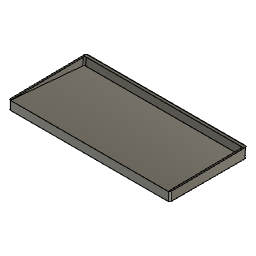
Resistor Stand v4 (Autodesk Fusion 360 design; units mm, degrees)
Autodesk Fusion 360 part; units mm, degrees
sketch "Sketch1" plane through (0, 0, 0) normal (1, 0, 0) x (0, 1, 0)
  line L0 (0, 0) -> (0, 5.5344)
  line L1 (0, 5.5344) -> (63.2584, 0)
  line L2 (63.2584, 0) -> (63.8118, 6.3258)
  line L3 (63.8118, 6.3258) -> (61.2815, 6.5472) construction
  line L4 (61.2815, 6.5472) -> (60.728, 0.2214) construction
  line L5 (0, 0) -> (63.2584, 0) construction
  line L6 (63.2584, 0) -> (63.2584, -1.905) construction
  line L7 (63.2584, -1.905) -> (0, -1.905)
  line L8 (0, -1.905) -> (0, 0)
  line L9 (66.3421, 6.1045) -> (65.7887, -0.2214)
  line L10 (63.8118, 6.3258) -> (66.3421, 6.1045) construction
  line L11 (63.2584, 0) -> (65.8081, 0) construction
  line L12 (65.8081, 0) -> (65.8081, -1.905)
  line L13 (65.8081, -1.905) -> (63.2584, -1.905)
  line L14 (63.8118, 6.3258) -> (66.3421, 6.1045) construction
  line L15 (63.8118, 6.3258) -> (66.3421, 6.3258)
  line L16 (66.3421, 6.3258) -> (66.3421, 6.1045)
  dimension "d1" = 2.54
  dimension "d3" = 6.35
  dimension "d4" = 63.5
  dimension "d7" = 1.905
  dimension "d15" = 5
  constraint coincident L0.start L5.start
  constraint vertical L0
  constraint perpendicular L1 L2
  constraint perpendicular L2 L3
  constraint coincident L1 L4.end
  constraint perpendicular L1 L4
  constraint horizontal L5
  constraint vertical L6
  constraint horizontal L7
  constraint vertical L8
  constraint symmetric L3.start L2 L10.start
  constraint symmetric L2 L3.end L9.start
  constraint symmetric L2 L4.end L9.end
  constraint coincident L9 L11.end
  constraint perpendicular L6 L11
  constraint perpendicular L11 L12
  constraint perpendicular L6 L13
  constraint horizontal L15
  constraint vertical L16
  measures "d1" distance of L2.end L3.end
  measures "d3" distance of L1.end L2.end
  measures "d4" distance of L0.end L1.end
  measures "d7" distance of L0.start L7.end
  measures "d15" angle of L1 L5
extrude "Extrude1" add sketch "Sketch1" along normal blind 135.255
sketch "Sketch2" plane through (135.255, 0, 0) normal (1, 0, 0) x (0, 1, 0)
  line L0 (65.8081, -1.905) -> (65.8081, 0)
  line L1 (65.8081, 0) -> (66.3421, 6.1045)
  line L2 (63.8118, 6.3258) -> (63.2584, 0)
  line L3 (63.2584, 0) -> (0, 5.5344)
  line L4 (0, 5.5344) -> (0, -1.905)
  line L5 (0, -1.905) -> (65.8081, -1.905)
  line L6 (63.8118, 6.3258) -> (0, 5.5344)
  line L7 (63.8118, 6.3258) -> (66.3421, 6.3572)
  line L8 (66.3421, 6.3572) -> (66.3421, 6.1045)
  line L9 (66.3421, 6.3258) -> (63.8118, 6.3258)
  line L10 (66.3421, 6.1045) -> (66.3421, 6.3258)
  constraint coincident L2.start L6.start
  constraint parallel L6 L7
  constraint coincident L1.end L8.end
  constraint vertical L8
  constraint coincident L3.end L4.start
extrude "Extrude2" add sketch "Sketch2" along normal blind 1.27 contours L0 L1 L2 L3 L4 L5 L8 L9 L10 | L2 L3 L6
extrude "Extrude3" add 1 faces at (136.525, 43.2066, 0.8386) along direction (-1, 0, 0) blind 1.27 from surface at 136.525
fillet "Fillet1" radius 1.27 8 edges at (0, 63.5351, 3.1629) (135.255, 63.5351, 3.1629) (-1.27, 66.0751, 3.0522) (-1.27, 65.8081, -0.9525) (136.525, 66.0751, 3.0522) (136.525, 65.8081, -0.9525) (-1.27, 0, 1.8147) (136.525, 0, 1.8147)
